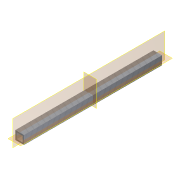
# Autodesk Inventor part: Lift Brace
Saved by Autodesk Inventor 2011 (Build 150239000, 239)
## iProperties
Created: 2014-09-14
Part Number: Lift Brace
Document SubType Name: Modeling
Designer: Family Room
Density: 1 g/cm^3
Author: Family Room
Autodesk Inventor part; units mm, degrees
ref_plane "YZ Plane" through (0, 0, 0) normal (1, 0, 0) x (0, 1, 0)
ref_plane "XZ Plane" through (0, 0, 0) normal (0, 1, 0) x (-1, 0, 0)
ref_plane "XY Plane" through (0, 0, 0) normal (0, 0, 1) x (1, 0, 0)
sketch "Sketch1" plane through (0, 0, 0) normal (0, 0, 1) x (1, 0, 0)
  line L0 (0, 0) -> (19.05, 0)
  line L1 (19.05, 0) -> (19.05, 19.05)
  line L2 (19.05, 19.05) -> (0, 19.05)
  line L3 (0, 19.05) -> (0, 0)
  line L4 (15.875, 15.875) -> (15.875, 3.175)
  line L5 (15.875, 3.175) -> (3.175, 3.175)
  line L6 (3.175, 3.175) -> (3.175, 15.875)
  line L7 (3.175, 15.875) -> (15.875, 15.875)
  dimension "d0" = 19.05
  dimension "d1" = 19.05
  dimension "d2" = 3.175
  constraints: 16 end point, 4 parallel, 2 perpendicular, 1 horizontal, 3 other
  measures "d0" distance of L2.end L1.end
  measures "d1" distance of L1.end L0.end
  measures "d2" distance between parallel lines of L3 L6
extrude "Extrusion1" add sketch "Sketch1" along normal blind 304.8
ref_plane "Work Plane1" through (0, 0, 152.4) normal (0, 0, 1) x (1, 0, 0)
ref_plane "Work Plane2" through (0, 9.525, 0) normal (0, 1, 0) x (1, 0, 0)
ref_plane "Work Plane3" through (9.525, 0, 0) normal (1, 0, 0) x (0, 0, -1)
body "Solid1"
